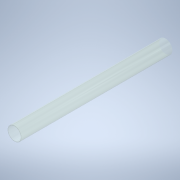
# Autodesk Inventor part: OuterGlassTube
Saved by Autodesk Inventor 2020 (Build 240168000, 168)
## iProperties
Created: 2019-09-29
Part Number: OuterGlassTube
Material: Glass
Document SubType Name: Modeling
Designer: vmiguel
Density: 2.18 g/cm^3
Appearance: Clear
Author: vmiguel
Autodesk Inventor part; units mm, degrees
ref_plane "YZ Plane" through (0, 0, 0) normal (1, 0, 0) x (0, 1, 0)
ref_plane "XZ Plane" through (0, 0, 0) normal (0, 1, 0) x (-1, 0, 0)
ref_plane "XY Plane" through (0, 0, 0) normal (0, 0, 1) x (1, 0, 0)
sketch "Sketch1" plane through (0, 0, 0) normal (0, 0, 1) x (1, 0, 0)
  circle A0 centre (0, 0) radius 21
  circle A1 centre (0, 0) radius 23
  dimension "d0" = 42
  dimension "d1" = 2
  constraints: 2 centre point, 1 coincident
  measures "d0" diameter of A0
  measures "d1" radial gap between concentric circles of A0 A1
extrude "Extrusion1" add sketch "Sketch1" against normal blind 500
body "Solid1"
